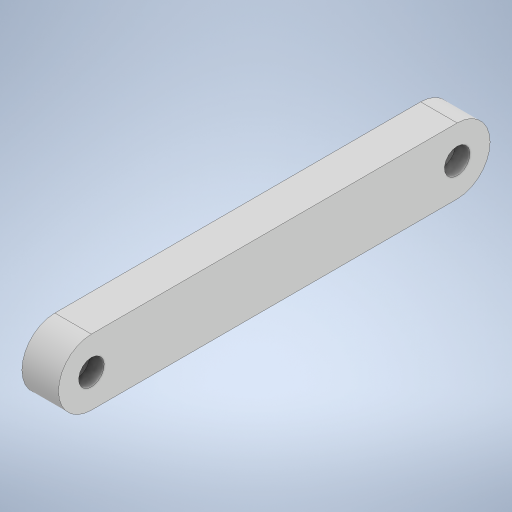
# Autodesk Inventor part: belka_2
Saved by Autodesk Inventor 2023 (Build 270158000, 158)
## iProperties
Created: 2024-05-12
Part Number: belka_2
Material: Ogólny
Document SubType Name: Modeling
Designer: kamil
Density: 1 g/cm^3
Appearance: Domyślna
Author: kamil
Autodesk Inventor part; units mm, degrees
ref_plane "YZ Plane" through (0, 0, 0) normal (1, 0, 0) x (0, 1, 0)
ref_plane "XZ Plane" through (0, 0, 0) normal (0, 1, 0) x (-1, 0, 0)
ref_plane "XY Plane" through (0, 0, 0) normal (0, 0, 1) x (1, 0, 0)
sketch "Szkic1" plane through (0, 0, 0) normal (1, 0, 0) x (0, 1, 0)
  line L0 (9.9771, 19.755) -> (9.9771, -30.245) construction
  line L1 (5.4771, 19.755) -> (5.4771, -30.245)
  line L2 (14.4771, -30.245) -> (14.4771, 19.755)
  arc A0 (14.4771, 19.755) -> (5.4771, 19.755) centre (9.9771, 19.755) ccw
  arc A1 (5.4771, -30.245) -> (14.4771, -30.245) centre (9.9771, -30.245) ccw
  circle A2 centre (9.9771, 19.755) radius 1.75
  circle A3 centre (9.9771, -30.245) radius 1.75
  point P0 (0, 0)
  point P1 (9.9771, -5.245)
  dimension "d0" = 50
  dimension "d1" = 9
  dimension "d2" = 3.5
  dimension "d3" = 3.5
  constraints: 8 end point, 4 centre point, 4 point on circle, 4 tangent, 2 coincident, 1 midpoint, 1 parallel, 1 vertical
  measures "d0" distance of L0.start L0.end
  measures "d1" diameter of A1
  measures "d2" diameter of A2
  measures "d3" diameter of A3
extrude "Wyciągnięcie proste1" add sketch "Szkic1" along normal blind 5
sketch "Szkic5" plane through (0, 0, 0) normal (-1, 0, 0) x (0, 0, 1)
  circle A0 centre (19.755, 9.9771) radius 1.75 projected
  circle A1 centre (-30.245, 9.9771) radius 1.75 projected
  circle A2 centre (19.755, 9.9771) radius 3
  circle A3 centre (-30.245, 9.9771) radius 3
  point P0 (0, 0)
  dimension "d20" = 6
  dimension "d21" = 6
  constraints: 2 centre point, 2 coincident
  measures "d20" diameter of A2
  measures "d21" diameter of A3
extrude "Wyciągnięcie proste6" cut sketch "Szkic5" against normal blind 3 contours A0 | A1 | A2 | A3
